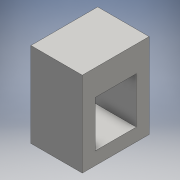
# Autodesk Inventor part: Syring Mount
Saved by Autodesk Inventor 2016 (Build 200138000, 138)
## iProperties
Created: 2016-05-08
Part Number: Syring Mount
Material: Generic
Document SubType Name: Modeling
Designer: Kenneth Daniel
Density: 1 g/cm^3
Appearance: Default
Author: Kenneth Daniel
Autodesk Inventor part; units mm, degrees
ref_plane "YZ Plane" through (0, 0, 0) normal (1, 0, 0) x (0, 1, 0)
ref_plane "XZ Plane" through (0, 0, 0) normal (0, 1, 0) x (-1, 0, 0)
ref_plane "XY Plane" through (0, 0, 0) normal (0, 0, 1) x (1, 0, 0)
sketch "Sketch1" plane through (0, 0, 0) normal (0, 1, 0) x (-1, 0, 0)
  line L0 (-10, 16.5) -> (10, 16.5)
  line L1 (10, 16.5) -> (10, -16.5)
  line L2 (10, -16.5) -> (-10, -16.5)
  line L3 (-10, -16.5) -> (-10, 16.5)
  line L4 (-10, 16.5) -> (10, -16.5) construction
  line L5 (10, 16.5) -> (-10, -16.5) construction
  point P0 (0, 0)
  dimension "d0" = 20
  dimension "d1" = 33
  constraints: 12 end point, 2 midpoint, 2 parallel, 1 horizontal, 1 perpendicular
  measures "d0" distance of L0.start L0.end
  measures "d1" distance of L0.end L1.end
extrude "Extrusion1" add sketch "Sketch1" along normal blind 26
sketch "Sketch2" plane through (10, 0, 16.5) normal (1, 0, 0) x (0, 0, -1)
  line L0 (0, 26) -> (33, 26) projected
  line L1 (0, 26) -> (0, 21)
  line L2 (0, 0) -> (0, 26) projected
  line L3 (10, 21) -> (28, 21)
  line L4 (33, 0) -> (33, 26) projected
  line L5 (33, 26) -> (28, 26)
  line L6 (28, 21) -> (28, 5)
  line L7 (33, 0) -> (0, 0) projected
  line L8 (33, 0) -> (33, 5)
  line L9 (28, 5) -> (10, 5)
  line L10 (0, 26) -> (10, 26)
  line L11 (10, 21) -> (10, 5)
  point P0 (16.5, 0)
  dimension "d4" = 5
  dimension "d5" = 5
  dimension "d6" = 5
  dimension "d7" = 10
  constraints: 16 end point, 4 perpendicular, 4 point on line
  measures "d4" distance of L0.start L1.end
  measures "d5" distance of L0.end L5.end
  measures "d6" distance of L4.start L8.end
  measures "d7" distance of L0.start L10.end
extrude "Extrusion2" cut sketch "Sketch2" against normal blind 26 contours L3 L6 L9 L11
body "Solid1"
